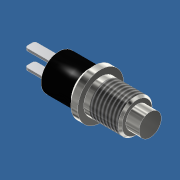
# Autodesk Inventor part: Bouton
Saved by Autodesk Inventor 2015 SP2 (Build 190223200, 223)
## iProperties
Created: 2017-10-30
Part Number: Bouton
Material: Générique
Document SubType Name: Modeling
Designer: Alexandre.PICOTTE
Density: 1 g/cm^3
Appearance: Par défaut
Author: Alexandre.PICOTTE
Autodesk Inventor part; units mm, degrees
ref_plane "YZ Plane" through (0, 0, 0) normal (1, 0, 0) x (0, 1, 0)
ref_plane "XZ Plane" through (0, 0, 0) normal (0, 1, 0) x (-1, 0, 0)
ref_plane "XY Plane" through (0, 0, 0) normal (0, 0, 1) x (1, 0, 0)
sketch "Esquisse1" plane through (0, 0, 0) normal (0, 0, 1) x (1, 0, 0)
  line L0 (-14.8768, 0) -> (-3.0909, 0)
  line L1 (0, 3.7) -> (0, 0)
  line L2 (8.6, 4.75) -> (7.2, 4.75)
  line L3 (8.6, 3.5) -> (8.6, 4.75)
  line L4 (8.6, 3.5) -> (16.1, 3.5)
  line L5 (16.1, 3.5) -> (16.1, 2.3)
  line L6 (16.1, 2.3) -> (18.8, 2.3)
  line L7 (18.8, 2.3) -> (18.8, 3)
  line L8 (0, 3.7) -> (6.2, 3.7)
  line L9 (6.2, 3.7) -> (7.2, 4.75)
  line L10 (18.8, 2.3) -> (18.8, 0)
  line L11 (18.8, 0) -> (0, 0)
  dimension "d4" = 9.5
  dimension "d5" = 7
  dimension "d6" = 4.6
  dimension "d9" = 1.4
  dimension "d10" = 7.4
  dimension "d11" = 1
  dimension "d12" = 7.5
  dimension "d15" = 2.7
  dimension "d16" = 18.8
  constraints: 24 end point, 5 horizontal, 3 perpendicular, 3 point on line, 2 vertical
  measures "d4" diameter of L2 L0
  measures "d5" diameter of L4 L0
  measures "d6" diameter of L6 L0
  measures "d9" distance of L2.start L2.end
  measures "d10" diameter of L8 L0
  measures "d11" horizontal distance of L2.end L8.end
  measures "d12" distance of L3.start L4.end
  measures "d15" distance of L5.end L6.end
  measures "d16" distance between parallel lines of L7 L1
revolve "Révolution1" add sketch "Esquisse1" angle 360 about axis through (-14.8768, 0, 0) along (1, 0, 0)
thread "Filetage1" size "M7x0.75" class "6g" standard "ANSI Metric M Profile" length 6.3
chamfer "Chanfrein1" distance 0.4 angle 45 1 edges at (16.1, -3.5, 0)
sketch "Esquisse2" plane through (0, 0, 0) normal (-1, 0, 0) x (0, 0, 1)
  line L0 (2, -1) -> (1.5, -1)
  line L1 (1.5, -1) -> (1.5, 1)
  line L2 (1.5, 1) -> (2, 1)
  line L3 (2, 1) -> (2, -1)
  line L4 (-1.5, -1) -> (-2, -1)
  line L5 (-2, -1) -> (-2, 1)
  line L6 (-2, 1) -> (-1.5, 1)
  line L7 (-1.5, 1) -> (-1.5, -1)
  line L8 (0, -6.65) -> (0, 6.65) construction
  line L9 (-6.65, 0) -> (6.65, 0) construction
  point P0 (0, 0)
  dimension "d23" = 0.5
  dimension "d24" = 2
  dimension "d25" = 3
  constraints: 16 end point, 4 parallel, 2 horizontal, 2 perpendicular, 5 other
  measures "d23" distance of L0.start L0.end
  measures "d24" distance of L2.end L0.start
  measures "d25" distance between parallel lines of L7 L1
extrude "Extrusion1" add sketch "Esquisse2" along normal blind 6
fillet "Congé1" radius 0.5 4 edges at (-6, -1, 1.75) (-6, 1, 1.75) (-6, 1, -1.75) (-6, -1, -1.75)
